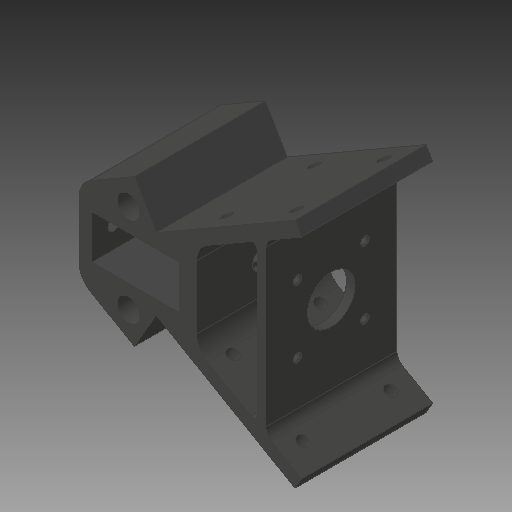
# Autodesk Inventor part: Coins inferieur
Saved by Autodesk Inventor 2017 (Build 210142000, 142)
## iProperties
Company: FABLAB Frenchmakers
Part Number: Coins inferieur
Material: Aluminium
Document SubType Name: Modeling
Designer: FABLAB Frenchmakers
Density: 2.7 g/cm^3
Appearance: Par défaut(1)
Mass: 417.6 g
Surface Area: 516.186 cm^2
Volume: 154.667 cm^3
Stock Number: 1420-01-05
Project: 1420 Vauban 3D XL
Catalog Web Link: http://frenchmakers.com/
Autodesk Inventor part; units mm, degrees
ref_plane "YZ Plane" through (0, 0, 0) normal (1, 0, 0) x (0, 1, 0)
ref_plane "XZ Plane" through (0, 0, 0) normal (0, 1, 0) x (-1, 0, 0)
ref_plane "XY Plane" through (0, 0, 0) normal (0, 0, 1) x (1, 0, 0)
sketch "Esquisse1" plane through (0, 0, 0) normal (0, 0, 1) x (1, 0, 0)
  line L0 (0, 0) -> (0, 38.6276)
  line L1 (0, 38.6276) -> (16.5, 48.1538)
  line L2 (16.5, 48.1538) -> (13.5, 53.35)
  line L3 (13.5, 53.35) -> (-50.3694, 16.475)
  line L4 (-50.3694, 16.475) -> (-60.3694, 33.7955)
  line L5 (-60.3694, 33.7955) -> (-80.7, 22.0576)
  line L6 (-85.7, 13.3974) -> (-85.7, 0)
  line L7 (-85.7, 0) -> (0, 0)
  arc A0 (-80.7, 22.0576) -> (-85.7, 13.3974) centre (-75.7, 13.3974) ccw
  line L8 (-79.9, 0) -> (-39.75, 0) construction
  line L9 (-39.75, 0) -> (-39.75, 10.075) construction
  line L10 (-39.75, 10.075) -> (-79.9, 10.075) construction
  line L11 (-79.9, 10.075) -> (-79.9, 0) construction
  dimension "d0" = 20
  dimension "d1" = 73.75
  dimension "d3" = 6
  dimension "d4" = 16.5
  dimension "d7" = 85.7
  dimension "d32" = 40.15
  dimension "d33" = 5.8
  dimension "d34" = 10.075
  dimension "d35" = 6.4
  dimension "d38" = 120
  dimension "d39" = 10
  constraints: 24 end point, 5 perpendicular, 4 parallel, 2 point on circle, 2 tangent, 1 centre point, 1 coincident, 1 horizontal, 1 point on line, 1 vertical
  measures "d0" distance of L3.end L4.end
  measures "d1" distance of L2.end L3.end
  measures "d3" distance of L1.end L2.end
  measures "d4" distance from line of L1.end L0
  measures "d7" distance between parallel lines of L0 L6
  measures "d32" distance of L9.end L10.end
  measures "d33" distance between parallel lines of L6 L11
  measures "d34" distance between parallel lines of L8 L10
  measures "d35" distance from line of L3.end L10
  measures "d38" angle of L5 L6
  measures "d39" radius of A0
extrude "Embase" add sketch "Esquisse1" along normal mid plane 60.3
mirror "Symétrie1" about plane through (-85.7, 0, 0) normal (0, -1, 0) of "Embase"
sketch "Esquisse2" plane through (0, 0, 30.15) normal (0, 0, 1) x (1, 0, 0)
  line L0 (-79.95, -10.075) -> (-39.8, -10.075)
  line L1 (-39.8, -10.075) -> (-39.8, 10.075)
  line L2 (-39.8, 10.075) -> (-79.95, 10.075)
  line L3 (-79.95, 10.075) -> (-79.95, -10.075)
  line L4 (0, 38.6276) -> (0, -38.6276) projected
  line L5 (-85.7, 13.3974) -> (-85.7, -13.3974) projected
  point P0 (0, 0)
  point P1 (-39.8, 0)
  point P2 (0, 0)
  dimension "d14" = 20.15
  dimension "d15" = 40.15
  dimension "d16" = 5.75
  constraints: 8 end point, 2 midpoint, 2 parallel, 1 horizontal, 1 horizontal alignment, 1 perpendicular
  measures "d14" distance of L0.end L1.end
  measures "d15" distance of L1.end L2.end
  measures "d16" distance between parallel lines of L5 L3
extrude "Passage profilé" cut sketch "Esquisse2" against normal through all
sketch "Esquisse3" plane through (0, 0, 30.15) normal (0, 0, 1) x (1, 0, 0)
  line L0 (-31.8, -20.3371) -> (-31.8, 20.3371)
  line L1 (-31.8, 20.3371) -> (-3.9, 36.4452)
  line L2 (-3.9, 36.4452) -> (-3.9, -36.4452)
  line L3 (-31.8, -20.3371) -> (-3.9, -36.4452)
  line L4 (0, 38.6276) -> (0, -38.6276) projected
  line L5 (13.5, 53.35) -> (-50.3694, 16.475) projected
  line L6 (13.5, -53.35) -> (-50.3694, -16.475) projected
  point P0 (0, 0)
  dimension "d19" = 27.9
  dimension "d20" = 3.9
  dimension "d21" = 5.94
  dimension "d22" = 5.94
  constraints: 8 end point, 2 parallel, 1 equal length, 1 vertical
  measures "d19" distance between parallel lines of L2 L0
  measures "d20" distance between parallel lines of L4 L2
  measures "d21" distance between parallel lines of L5 L1
  measures "d22" distance between parallel lines of L6 L3
extrude "Passage courroie" cut sketch "Esquisse3" against normal through all
fillet "Congé1" radius 10 2 edges at (-31.8, -20.3371, 0) (-31.8, 20.3371, 0)
fillet "Congé1" radius 2 2 edges at (-3.9, 36.4452, 0) (-3.9, -36.4452, 0)
fillet "Congé1" radius 5 2 edges at (0, 38.6276, 0) (0, -38.6276, 0)
sketch "Esquisse7" plane through (0, 0, 30.15) normal (0, 0, 1) x (1, 0, 0)
  point P0 (0, 0)
  point P1 (-63, -20.5)
  point P2 (-63, 20.5)
  dimension "d51" = 20.5
  dimension "d52" = 63
  dimension "d53" = 20.5
  dimension "d54" = 63
  measures "d51" vertical distance of point (0, 0) point (-63, -20.5)
  measures "d52" horizontal distance of point (0, 0) point (-63, -20.5)
  measures "d53" vertical distance of point (0, 0) point (-63, 20.5)
  measures "d54" horizontal distance of point (0, 0) point (-63, 20.5)
hole "Perçage axe" at (-63, -20.5, 30.15) at (-63, 20.5, 30.15) direction (0, 0, -1) diameter 10.5 end through all
sketch "Esquisse8" plane through (13.5, -53.35, -30.15) normal (-0.5, -0.8660254, 0) x (0.8660254, -0.5, 0)
  line L0 (0, 60.3) -> (0, 0) projected
  line L1 (-73.75, 0) -> (0, 0) projected
  line L2 (0, 60.3) -> (-73.75, 60.3) projected
  point P0 (-38.3663, 30.15)
  point P1 (-47.9, 10)
  point P2 (-47.9, 50.3)
  point P3 (-10.8, 10)
  point P4 (-10.8, 50.3)
  dimension "d55" = 10.8
  dimension "d56" = 37.1
  dimension "d57" = 10
  dimension "d58" = 10
  constraints: 2 horizontal alignment, 2 vertical alignment
  measures "d55" distance from line of L0 point (-10.8, 50.3)
  measures "d56" distance of point (-10.8, 50.3) point (-47.9, 50.3)
  measures "d57" distance from line of L1 point (-10.8, 10)
  measures "d58" distance from line of L2 point (-10.8, 50.3)
hole "Maintient profilé horizontal" at (-27.9826, -29.4, -20.15) at (-27.9826, -29.4, 20.15) at (4.1469, -47.95, -20.15) at (4.1469, -47.95, 20.15) direction (0.5, 0.8660254, 0) diameter 5.1 depth 8 tip angle 118
mirror "Symétrie2" about plane through (0, 0, 0) normal (0, 1, 0) of "Maintient profilé horizontal"
sketch "Esquisse9" plane through (0, -35.7408, 30.15) normal (1, 0, 0) x (0, 0, -1)
  point P0 (30.15, 35.7408)
  point P1 (30.15, 35.7408)
  constraints: 1 coincident
hole "Passage moteur + poulie" at (0, 0, 0) direction (-1, 0, 0) diameter 21.9 depth 8 tip angle 118
sketch "Esquisse10" plane through (0, -35.7408, 30.15) normal (1, 0, 0) x (0, 0, -1)
  point P0 (30.15, 35.7408)
  point P1 (14.65, 20.2408)
  point P2 (45.65, 20.2408)
  point P3 (45.65, 51.2408)
  point P4 (14.65, 51.2408)
  dimension "d73" = 31
  dimension "d74" = 31
  dimension "d75" = 15.5
  dimension "d76" = 15.5
  constraints: 2 horizontal alignment, 2 vertical alignment
  measures "d73" distance of point (14.65, 51.241) point (14.65, 20.241)
  measures "d74" distance of point (45.65, 51.241) point (14.65, 51.241)
  measures "d75" horizontal distance of point (14.65, 51.241) point (30.15, 35.741)
  measures "d76" horizontal distance of point (14.65, 51.241) point (30.15, 35.741)
hole "Maintient moteur" at (0, -15.5, 15.5) at (0, -15.5, -15.5) at (0, 15.5, -15.5) at (0, 15.5, 15.5) direction (-1, 0, 0) diameter 3 depth 8 tip angle 118 countersink diameter 4 countersink angle 90
sketch "Esquisse11" plane through (-31.8, -14.5636, 30.15) normal (1, 0, 0) x (0, 0, -1)
  point P0 (30.15, 14.5636)
  point P1 (30.15, 14.5636)
  constraints: 1 coincident
hole "Perçage5" at (-31.8, 0, 0) direction (-1, 0, 0) diameter 5 depth 8 tip angle 118 counterbore diameter 8.75 counterbore depth 3
sketch "Esquisse12" plane through (-85.7, 13.3974, -30.15) normal (-1, 0, 0) x (0, 0, 1)
  point P0 (30.15, -13.3974)
  point P1 (10.15, -13.3974)
  point P2 (50.15, -13.3974)
  dimension "d91" = 40
  dimension "d92" = 20
  constraints: 2 horizontal alignment
  measures "d91" distance of point (50.15, -13.397) point (10.15, -13.397)
  measures "d92" distance of point (30.15, -13.397) point (50.15, -13.397)
hole "Maintient profilé vertical" at (-85.7, 0, -20) at (-85.7, 0, 20) direction (1, 0, 0) diameter 5.5 depth 8 tip angle 118 countersink diameter 10 countersink angle 90
equation "\"d22\" = d21"
equation "\"d53\" = d51"
equation "\"d54\" = d52"
equation "\"d75\" = 0.5 * d73"
equation "\"d76\" = 0.5 * d74"
equation "\"d92\" = 0.5 * d91"
